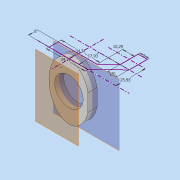
# Autodesk Inventor part: lw_4_крепление
Saved by Autodesk Inventor 2019 (Build 230136000, 136)
## iProperties
Created: 2021-03-07
Part Number: lw_4_крепление
Material: Типовые
Document SubType Name: Modeling
Designer: Kurbatova
Density: 1 g/cm^3
Appearance: По умолчанию
Author: Kurbatova
Autodesk Inventor part; units mm, degrees
ref_plane "YZ Plane" through (0, 0, 0) normal (1, 0, 0) x (0, 1, 0)
ref_plane "XZ Plane" through (0, 0, 0) normal (0, 1, 0) x (-1, 0, 0)
sketch "Эскиз1" plane through (0, 0, 0) normal (0, 1, 0) x (-1, 0, 0)
  line L0 (21.0127, -18.1102) -> (-13.2973, -18.1102)
  line L1 (21.0127, -18.1102) -> (21.0127, -10.1102)
  line L2 (21.0127, -10.1102) -> (-13.2973, -10.1102)
  line L3 (20.451, -28.0402) -> (-43.6243, -28.0402)
  line L4 (-23.5473, -28.0402) -> (-23.5473, -44.0402)
  line L5 (-23.5473, -44.0402) -> (-31.5473, -44.0402)
  line L6 (-31.5473, -44.0402) -> (-31.5473, -28.0402)
  line L7 (-31.5473, -28.0402) -> (-13.2973, -10.1102)
  line L8 (-23.5473, -28.0402) -> (-13.2973, -18.1102)
  line L9 (-5.2293, -36.0402) -> (-38.0765, -36.0402)
  line L10 (31.3847, -10.1102) -> (-49.5844, -10.1102)
  line L11 (3.1555, -40.2525) -> (3.1555, 5.5167)
  point P0 (0, 0)
  point P1 (-23.5473, -36.0402)
  dimension "d0" = 34.31
  dimension "d2" = 8
  dimension "d3" = 34.31
  dimension "d5" = 8
  dimension "d7" = 17.93
  dimension "d8" = 25.93
  dimension "d9" = 10.25
  dimension "d10" = 8
  constraints: 24 end point, 4 perpendicular, 4 point on line, 3 horizontal, 3 vertical, 1 midpoint
  measures "d0" distance of L0.start L0.end
  measures "d2" distance of L0.start L1.end
  measures "d3" distance of L1.end L2.end
  measures "d5" distance of L4.end L5.end
  measures "d7" vertical distance of L6.end L2.end
  measures "d8" distance between parallel lines of L10 L9
  measures "d9" distance from line of L0.end L4
  measures "d10" distance of L6.end L4.start
extrude "Выдавливание1" add sketch "Эскиз1" against normal blind 49.99 contours L0 L11 L2 L1 | L0 L8 L3 L7 L2 L11 | L4 L9 L6 L3 | L4 L5 L6 L9
ref_plane "РабПлоскость4" through (13.2973, 0, -14.1102) normal (0, 0, -1) x (-1, 0, 0)
sketch "Эскиз7" plane through (13.2973, 0, -18.1102) normal (0, 0, -1) x (-1, 0, 0)
  line L0 (0, 0) -> (0, -49.99) projected
  line L1 (17.155, -59.5912) -> (17.155, 20.4726)
  line L2 (47.8268, -24.995) -> (-14.3296, -24.995)
  line L3 (0, 0) -> (34.31, 0) projected
  line L4 (34.31, -49.99) -> (0, -49.99) projected
  ellipse E0 centre (16.7486, -24.995) end of major axis (34.3073, -25.2131) minor radius 24.9985 (0, -32.7251) -> (0, -17.692) ccw
  line L5 (34.31, 0) -> (34.31, -49.99) projected
  circle A0 centre (16.7486, -24.995) radius 12.5
  ellipse E1 centre (16.7486, -24.995) end of major axis (34.3073, -25.2131) minor radius 24.9985 (0, -32.7251) -> (16.3422, -49.99) ccw
  point P0 (0, -24.995)
  point P1 (17.155, 0)
  dimension "d29" = 17.56
  dimension "d31" = 25
  constraints: 5 point on line, 4 end point, 3 midpoint, 2 vertical, 1 centre point, 1 coincident, 1 horizontal, 9 other
  measures "d31" diameter of A0
extrude "Выдавливание2" cut sketch "Эскиз7" against normal blind 45 contours E0 L3 L1 A0 L2 L0 | L2 A0 L1 E0 L4 L0 | E0 L2 A0 L1 | A0 L2 E0 L1 keep common part
